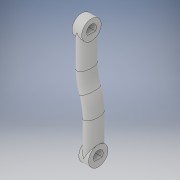
# Autodesk Inventor part: Рукоядь
Saved by Autodesk Inventor 2019 (Build 230136000, 136)
## iProperties
Created: 2019-04-27
Part Number: Рукоядь
Material: Типовые
Document SubType Name: Modeling
Designer: BarmanKaktus
Density: 1 g/cm^3
Appearance: По умолчанию
Author: BarmanKaktus
Autodesk Inventor part; units mm, degrees
ref_plane "YZ Plane" through (0, 0, 0) normal (1, 0, 0) x (0, 1, 0)
sketch "Эскиз6" plane through (0, 0, 0) normal (0, 0, 1) x (1, 0, 0)
  line L0 (0, 0) -> (0, 34.1571)
  line L1 (-7, 74.5427) -> (-7, 108.735)
  arc A0 (-7, 74.5427) -> (-3.5, 54.3499) centre (53, 74.5427) ccw
  arc A1 (0, 34.1571) -> (-3.5, 54.3499) centre (-60, 34.1571) ccw
  point P0 (0, 45)
  point P1 (-7, 63.735)
  dimension "d20" = 45
  dimension "d22" = 45
  dimension "d23" = 7
  dimension "d24" = 60
  constraints: 4 end point, 4 point on circle, 3 tangent, 2 centre point, 2 point on line, 1 equal radius, 1 parallel, 1 vertical
  measures "d20" distance of L0.start point (0, 45)
  measures "d22" distance of point (-7, 63.735) L1.end
  measures "d23" horizontal distance of point (0, 45) point (-7, 63.735)
  measures "d24" radius of A0
ref_plane "РабПлоскость5" through (0, 0, 0) normal (0, 1, 0) x (-1, 0, 0)
sketch "Эскиз12" plane through (0, 0, 0) normal (0, 1, 0) x (-1, 0, 0)
  ellipse E0 centre (0, 0) end of major axis (5, 0) minor radius 10
  dimension "d35" = 5
  dimension "d36" = 10
  constraints: 1 coincident, 2 other
ref_plane "РабПлоскость6" through (-7, 108.735, 0) normal (0, 1, 0) x (-1, 0, 0)
sketch "Эскиз13" plane through (-7, 108.735, 0) normal (0, 1, 0) x (-1, 0, 0)
  ellipse E0 centre (0, 0) end of major axis (5, 0) minor radius 10
  point P0 (-7, 0)
  dimension "d37" = 5
  dimension "d38" = 10
  constraints: 2 other
sweep "Сдвиг1" add profiles "Эскиз12" path "Эскиз6"
ref_plane "РабПлоскость8" through (0, 0, 0) normal (0, -1, 0) x (1, 0, 0)
sketch "Эскиз16" plane through (0, 0, 0) normal (0, -1, 0) x (1, 0, 0)
  line L0 (-5, 10) -> (5, 10)
  line L1 (5, 10) -> (5, 0)
  line L2 (5, 0) -> (-5, 0)
  line L3 (-5, 0) -> (-5, 10)
  line L4 (-5, 10) -> (-5, 0)
  point P0 (0, 0)
  dimension "d46" = 10
  dimension "d47" = 10
  dimension "d54" = 5
  dimension "d55" = 10
  constraints: 10 end point, 3 equal length, 1 horizontal, 1 perpendicular
  measures "d46" distance of L1.end L2.end
  measures "d47" distance of L0.end L1.end
  measures "d54" distance from line of point (0, 0) L1
  measures "d55" distance from line of point (0, 0) L0
revolve "Вращение2" add sketch "Эскиз16" angle 360 about axis through (5, 0, 0) along (-1, 0, 0)
ref_plane "РабПлоскость9" through (-5, 0, 10) normal (0, 0, 1) x (1, 0, 0)
sketch "Эскиз17" plane through (-5, 0, 10) normal (0, 0, 1) x (1, 0, 0)
  circle A0 centre (5, 0) radius 5
  line L0 (2, -4) -> (2, 4)
  dimension "d50" = 10
  dimension "d51" = 3
  constraints: 2 end point, 2 point on circle, 1 centre point, 1 coincident, 1 vertical
  measures "d50" diameter of A0
  measures "d51" horizontal distance of point (5, 0) L0.start
extrude "Выдавливание1" [suppressed]
sketch "Эскиз18" plane through (-5, 0, 0) normal (-1, 0, 0) x (0, 0, 1)
  circle A0 centre (0, 0) radius 5
  line L0 (4, -3) -> (-4, -3)
  dimension "d56" = 10
  dimension "d57" = 3
  constraints: 2 end point, 2 point on circle, 1 centre point, 1 coincident, 1 horizontal
  measures "d56" diameter of A0
  measures "d57" distance from line of L0 point (0, 0)
extrude "Выдавливание2" cut sketch "Эскиз18" against normal through all contours A0 L0 picked at (1.1374, 0.1102)
sketch "Эскиз19" plane through (-7, 108.735, 0) normal (0, 1, 0) x (1, 0, 0)
  line L0 (-1.2083, 0) -> (-5, 0) projected
  line L1 (-5, 0) -> (5, 0)
  line L2 (5, 0) -> (5, 10)
  line L3 (5, 10) -> (-5, 10)
  line L4 (-5, 10) -> (-5, 0)
  point P0 (7, 0)
  dimension "d60" = 10
  dimension "d61" = 10
  constraints: 8 end point, 2 parallel, 1 horizontal, 1 perpendicular
  measures "d60" distance of L2.end L3.end
  measures "d61" distance of L1.end L2.end
revolve "Вращение3" add sketch "Эскиз19" angle 360 about axis through (-12, 108.735, 0) along (1, 0, 0)
sketch "Эскиз20" plane through (-12, 108.735, 0) normal (-1, 0, 0) x (0, 0, 1)
  circle A0 centre (0, 0) radius 5
  line L0 (4, -3) -> (-4, -3)
  point P0 (0, -108.735)
  dimension "d63" = 10
  constraints: 2 end point, 2 point on circle, 1 centre point, 1 horizontal
  measures "d63" diameter of A0
extrude "Выдавливание3" cut sketch "Эскиз20" against normal blind 50 contours A0 L0 picked at (1.1374, 0.1102)
